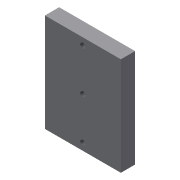
# Autodesk Inventor part: Sideplate
Saved by Autodesk Inventor 2022 (Build 260148000, 148)
## iProperties
Shininess: 64.0
Length Units: 11272
Angle Units: 11279
Time Units: 11290
Mass Units: 11286
Length Display Precision: 3
Angle Display Precision: 2
Compacted: True
Part Number: Sideplate
Document SubType Name: Modeling
Created: 2003-04-07
Designer: demo
Density: 1 g/cm^3
Material: Generic
Appearance: Default
Density: 0.0
Volumn: 0.0
Area: 0.0
PropertySet Name: Model Information
Control State: 0
Master: False
Checked Out: False
Author: demo
Autodesk Inventor part; units mm, degrees
ref_plane "YZ Plane" through (0, 0, 0) normal (1, 0, 0) x (0, 1, 0)
ref_plane "XZ Plane" through (0, 0, 0) normal (0, 1, 0) x (-1, 0, 0)
sketch "Sketch1" plane through (0, 0, 0) normal (0, 0, 1) x (1, 0, 0)
  line L0 (-14.4788, 22.2008) -> (188.7212, 22.2008)
  line L1 (188.7212, 22.2008) -> (188.7212, -240.6892)
  line L2 (188.7212, -240.6892) -> (-14.4788, -240.6892)
  line L3 (-14.4788, -240.6892) -> (-14.4788, 22.2008)
  dimension "d0" = 203.2
  dimension "d1" = 262.89
  constraints: 8 end point, 2 parallel, 1 horizontal, 1 perpendicular
  measures "d0" distance of L0.start L0.end
  measures "d1" distance of L2.end L0.start
extrude "Extrusion1" add sketch "Sketch1" along normal blind 38.1
sketch "Sketch2" plane through (0, 0, 38.1) normal (0, 0, 1) x (1, 0, 0)
  line L0 (188.7212, 22.2008) -> (188.7212, -240.6892) projected
  line L1 (-14.4788, 22.2008) -> (188.7212, 22.2008) projected
  point P0 (87.1212, -109.2442)
  dimension "d4" = 101.6
  dimension "d5" = 131.445
  measures "d4" distance from line of L0 point (87.121, -109.244)
  measures "d5" distance from line of L1 point (87.121, -109.244)
hole "Hole1" at (87.1212, -109.2442, 38.1) direction (0, 0, -1) diameter 13.3858 end through all thread size "5/8-11 UNC" class "1B" standard "ANSI Unified Screw Threads"
sketch "Sketch3" plane through (0, 0, 38.1) normal (0, 0, 1) x (1, 0, 0)
  circle A0 centre (87.1212, -109.2442) radius 6.6929 projected
  point P0 (87.1212, 3.2016)
  point P1 (87.1212, -221.69)
  dimension "d13" = 112.4458
  dimension "d14" = 112.4458
  measures "d13" distance of A0.centre point (87.121, -221.69)
  measures "d14" distance of point (87.121, 3.202) A0.centre
hole "Hole2" at (87.1212, 3.2016, 38.1) at (87.1212, -221.69, 38.1) direction (0, 0, -1) diameter 13.3858 end through all thread size "5/8-11 UNC" class "1B" standard "ANSI Unified Screw Threads"
ref_plane "Work Plane1" through (87.1212, -240.6892, 0) normal (1, 0, 0) x (0, 0, -1)
body "Solid1"
